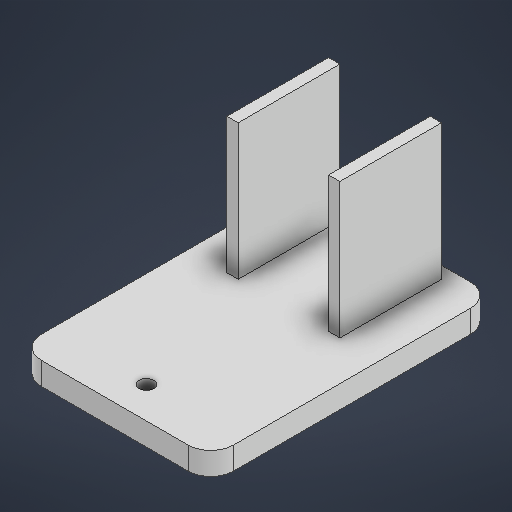
# Autodesk Inventor part: Camera Mount
Saved by Autodesk Inventor 2025 (Build 290162000, 162)
## iProperties
Created: 2024-10-25
Part Number: Camera Mount
Material: Generic
Document SubType Name: Modeling
Designer: mayhe
Density: 1 g/cm^3
Appearance: Default
Author: mayhe
Autodesk Inventor part; units mm, degrees
ref_plane "YZ Plane" through (0, 0, 0) normal (1, 0, 0) x (0, 1, 0)
ref_plane "XZ Plane" through (0, 0, 0) normal (0, 1, 0) x (-1, 0, 0)
ref_plane "XY Plane" through (0, 0, 0) normal (0, 0, 1) x (1, 0, 0)
sketch "Sketch6" plane through (0, 0, 0) normal (0, 1, 0) x (-1, 0, 0)
  line L0 (32.5, 62.5) -> (-32.5, 62.5)
  line L1 (-42.5, 52.5) -> (-42.5, -52.5)
  line L2 (-32.5, -62.5) -> (32.5, -62.5)
  line L3 (42.5, -52.5) -> (42.5, 52.5)
  line L4 (42.5, 62.5) -> (-42.5, -62.5) construction
  line L5 (-42.5, 62.5) -> (42.5, -62.5) construction
  circle A0 centre (0, -36.5125) radius 3.25
  circle A1 centre (0, 48.4875) radius 3.25
  arc A2 (32.5, -62.5) -> (42.5, -52.5) centre (32.5, -52.5) ccw
  arc A3 (-42.5, -52.5) -> (-32.5, -62.5) centre (-32.5, -52.5) ccw
  arc A4 (-32.5, 62.5) -> (-42.5, 52.5) centre (-32.5, 52.5) ccw
  arc A5 (42.5, 52.5) -> (32.5, 62.5) centre (32.5, 52.5) ccw
  circle A6 centre (0, 48.4875) radius 5.5
  circle A7 centre (0, -36.5125) radius 5.5
  line L6 (-1.445, 54.6718) -> (4.6332, 52.8311)
  line L7 (4.6332, 52.8311) -> (6.0782, 46.6468)
  line L8 (6.0782, 46.6468) -> (1.445, 42.3032)
  line L9 (1.445, 42.3032) -> (-4.6332, 44.1439)
  line L10 (-4.6332, 44.1439) -> (-6.0782, 50.3282)
  line L11 (-6.0782, 50.3282) -> (-1.445, 54.6718)
  line L12 (-1.445, -30.3282) -> (4.6332, -32.1689)
  line L13 (4.6332, -32.1689) -> (6.0782, -38.3532)
  line L14 (6.0782, -38.3532) -> (1.445, -42.6968)
  line L15 (1.445, -42.6968) -> (-4.6332, -40.8561)
  line L16 (-4.6332, -40.8561) -> (-6.0782, -34.6718)
  line L17 (-6.0782, -34.6718) -> (-1.445, -30.3282)
  point P0 (0, 0)
  point P1 (-3.7616, 52.5)
  point P2 (-3.7616, -32.5)
  dimension "d48" = 11
  dimension "d49" = 11
  dimension "d42" = 85
  dimension "d43" = 125
  dimension "d44" = 6.5
  dimension "d45" = 6.5
  dimension "d46" = 85
  dimension "d47" = 10
  constraints: 36 end point, 8 point on circle, 8 point on line, 8 tangent, 6 centre point, 4 coincident, 4 midpoint, 3 equal radius, 2 parallel, 1 horizontal, 1 perpendicular, 32 other
  measures "d42" distance of L5.end L4.end
  measures "d43" distance of L4.end L5.start
  measures "d44" diameter of A0
  measures "d45" diameter of A1
  measures "d46" distance of A1.centre A0.centre
  measures "d47" radius of A2
extrude "Extrusion6" add sketch "Sketch6" along normal blind 2 contours A5 L3 A2 L2 A3 L1 A4 L0 | A6 | A6 L7 L8 | A6 L6 L7 | L8 L9 A6 | A6 L11 L6 | L9 L10 A6 | A6 L10 L11 | A7 | A7 L13 L14 | A7 L12 L13 | L14 L15 A7 | A7 L17 L12 | L15 L16 A7 | A7 L16 L17
sketch "Sketch7" plane through (0, 2, 0) normal (0, 1, 0) x (1, 0, 0)
  circle A0 centre (0, -48.4875) radius 3.25 projected
  circle A1 centre (0, -48.4875) radius 5.5
  circle A2 centre (0, 36.5125) radius 3.25 projected
  circle A3 centre (0, 36.5125) radius 5.5
  line L0 (5.5, -51.6629) -> (0, -54.8384)
  line L1 (0, -54.8384) -> (-5.5, -51.6629)
  line L2 (-5.5, -51.6629) -> (-5.5, -45.3121)
  line L3 (-5.5, -45.3121) -> (0, -42.1366)
  line L4 (0, -42.1366) -> (5.5, -45.3121)
  line L5 (5.5, -45.3121) -> (5.5, -51.6629)
  line L6 (5.5, 33.3371) -> (0, 30.1616)
  line L7 (0, 30.1616) -> (-5.5, 33.3371)
  line L8 (-5.5, 33.3371) -> (-5.5, 39.6879)
  line L9 (-5.5, 39.6879) -> (0, 42.8634)
  line L10 (0, 42.8634) -> (5.5, 39.6879)
  line L11 (5.5, 39.6879) -> (5.5, 33.3371)
  line L12 (-32.5, 62.5) -> (32.5, 62.5)
  line L13 (42.5, 52.5) -> (42.5, -52.5)
  line L14 (32.5, -62.5) -> (-32.5, -62.5)
  line L15 (-42.5, -52.5) -> (-42.5, 52.5)
  line L16 (-42.5, 62.5) -> (42.5, -62.5) construction
  line L17 (42.5, 62.5) -> (-42.5, -62.5) construction
  arc A4 (-42.5, -52.5) -> (-32.5, -62.5) centre (-32.5, -52.5) ccw
  arc A5 (-32.5, 62.5) -> (-42.5, 52.5) centre (-32.5, 52.5) ccw
  arc A6 (42.5, 52.5) -> (32.5, 62.5) centre (32.5, 52.5) ccw
  arc A7 (32.5, -62.5) -> (42.5, -52.5) centre (32.5, -52.5) ccw
  point P0 (0, 0)
  point P1 (5.5, -48.4875)
  point P2 (5.5, 36.5125)
  dimension "d52" = 11
  dimension "d53" = 11
  dimension "d54" = 125
  dimension "d61" = 10
  constraints: 36 end point, 9 point on line, 8 point on circle, 8 tangent, 4 centre point, 4 coincident, 4 midpoint, 3 equal radius, 2 horizontal alignment, 2 parallel, 1 horizontal, 1 perpendicular, 30 other
  measures "d54" distance of L17.start L16.end
  measures "d61" radius of A4
extrude "Extrusion7" add sketch "Sketch7" along normal blind 3.125 contours L12 A6 L13 A7 L14 A4 L15 A5
sketch "Sketch8" plane through (0, 5.125, 0) normal (0, 1, 0) x (1, 0, 0)
  circle A0 centre (0, -48.4875) radius 3.25 projected
  circle A1 centre (0, -48.4875) radius 3.25
  circle A2 centre (0, 36.5125) radius 3.25 projected
  circle A3 centre (0, 36.5125) radius 3.25
  line L0 (-32.5, 62.5) -> (32.5, 62.5)
  line L1 (42.5, 52.5) -> (42.5, -52.5)
  line L2 (32.5, -62.5) -> (-32.5, -62.5)
  line L3 (-42.5, -52.5) -> (-42.5, 52.5)
  line L4 (-42.5, 62.5) -> (42.5, -62.5) construction
  line L5 (42.5, 62.5) -> (-42.5, -62.5) construction
  arc A4 (32.5, -62.5) -> (42.5, -52.5) centre (32.5, -52.5) ccw
  arc A5 (42.5, 52.5) -> (32.5, 62.5) centre (32.5, 52.5) ccw
  arc A6 (-32.5, 62.5) -> (-42.5, 52.5) centre (-32.5, 52.5) ccw
  arc A7 (-42.5, -52.5) -> (-32.5, -62.5) centre (-32.5, -52.5) ccw
  point P0 (0, 0)
  dimension "d62" = 10
  constraints: 12 end point, 8 point on circle, 8 point on line, 8 tangent, 6 centre point, 3 equal radius, 2 coincident, 2 midpoint, 2 parallel, 1 horizontal, 1 perpendicular
  measures "d62" radius of A4
extrude "Extrusion8" add sketch "Sketch8" along normal blind 4.875
sketch "Sketch9" plane through (0, 10, 0) normal (0, 1, 0) x (1, 0, 0)
  line L0 (0, -62.5) -> (0, 62.5)
  line L1 (32.5, 62.5) -> (-32.5, 62.5) projected
  line L2 (-25, 57.15) -> (-20, 57.15)
  line L3 (-20, 57.15) -> (-20, 12.15)
  line L4 (-20, 12.15) -> (-25, 12.15)
  line L5 (-25, 12.15) -> (-25, 57.15)
  line L6 (32.5, 62.5) -> (-32.5, 62.5) projected
  line L7 (25, 57.15) -> (20, 57.15)
  line L8 (20, 57.15) -> (20, 12.15)
  line L9 (20, 12.15) -> (25, 12.15)
  line L10 (25, 12.15) -> (25, 57.15)
  point P0 (0, 0)
  dimension "d65" = 5
  dimension "d66" = 45
  dimension "d67" = 20
  constraints: 18 end point, 4 symmetric about line, 2 midpoint, 2 parallel, 1 horizontal, 1 perpendicular
  measures "d65" distance of L3.end L4.end
  measures "d66" distance of L2.end L3.end
  measures "d67" horizontal distance of point (0, 62.5) L2.end
extrude "Extrusion9" add sketch "Sketch9" along normal blind 60
body "Solid2"
